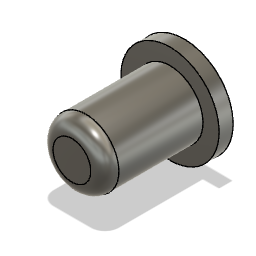
button (Autodesk Fusion 360 design; units mm, degrees)
Autodesk Fusion 360 part; units mm, degrees
sketch "Sketch1" plane through (0, 0, 6.57) normal (0, 0, 1) x (1, 0, 0)
  circle A0 centre (8.5, 8.89) radius 3.0492
  circle A1 centre (8.5, 8.89) radius 2.35
  dimension "d62" = 4.7
  dimension "d69" = 0
  dimension "d70" = 0
  dimension "d71" = 0
  dimension "d72" = 0
  dimension "d227" = 0
  dimension "d228" = 0
  dimension "d229" = 0
  dimension "d230" = 0
  dimension "d239" = 0
  dimension "d240" = 0
  dimension "d241" = 0
  dimension "d242" = 0
  dimension "d251" = 0
  dimension "d252" = 0
  dimension "d253" = 0
  dimension "d254" = 0
  dimension "d263" = 0
  dimension "d264" = 0
  dimension "d265" = 0
  dimension "d266" = 0
  dimension "d275" = 0
  dimension "d276" = 0
  dimension "d277" = 0
  dimension "d278" = 0
  dimension "d287" = 0
  dimension "d288" = 0
  dimension "d289" = 0
  dimension "d290" = 0
  dimension "d299" = 0
  dimension "d300" = 0
  dimension "d301" = 0
  dimension "d302" = 0
  dimension "d311" = 0
  dimension "d312" = 0
  dimension "d313" = 0
  dimension "d314" = 0
  dimension "d323" = 0
  dimension "d324" = 0
  dimension "d325" = 0
  dimension "d326" = 0
  constraint concentric A0 A1
  measures "d62" diameter of A1
extrude "Extrude1" add sketch "Sketch1" along normal blind 7 contours A1
sketch "Sketch2" plane through (0, 0, 6.57) normal (0, 0, -1) x (-1, 0, 0)
  circle A0 centre (-8.5, 8.89) radius 2.35
  circle A1 centre (-8.5, 8.89) radius 3.5
  dimension "d65" = 7
  constraint concentric A0 A1
  measures "d65" diameter of A1
extrude "Extrude2" add sketch "Sketch2" along normal blind 1 contours A0 | A1
fillet "Fillet1" radius 1 1 edges at (6.309, 8.0402, 13.57)
